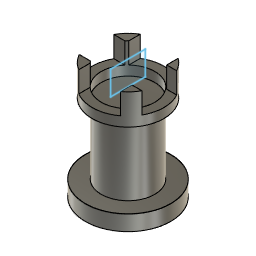
Rook v1 (Autodesk Fusion 360 design; units mm, degrees)
Autodesk Fusion 360 part; units mm, degrees
sketch "Sketch1" plane through (0, 0, 0) normal (0, 0, 1) x (1, 0, 0)
  circle A0 centre (0, 0) radius 27.94
  dimension "d1" = 55.88
  constraint coincident A0.centre origin
  measures "d1" diameter of A0
extrude "Extrude1" add sketch "Sketch1" along normal blind 10.16 makes body 1
sketch "Sketch2" plane through (0, 0, 0) normal (0, 0, 1) x (1, 0, 0)
  circle A0 centre (0, 0) radius 27.94
  dimension "d4" = 55.88
  constraint coincident A0.centre origin
  measures "d4" diameter of A0
extrude "Extrude2" add sketch "Sketch2" along normal blind 10 separate body makes body 2
sketch "Sketch3" plane through (0, 0, 10.16) normal (0, 0, 1) x (-1, 0, 0)
  circle A0 centre (0, 0) radius 27.94
  circle A1 centre (0, 0) radius 17.5
  dimension "d7" = 35
  constraint coincident A0.centre A1.centre
  measures "d7" diameter of A1
extrude "Extrude3" add sketch "Sketch3" along normal blind 46 contours A1 bodies 1
sketch "Sketch4" plane through (0, 0, 56.16) normal (0, 0, 1) x (-1, 0, 0)
  circle A0 centre (0, 0) radius 17.5
  circle A1 centre (0, 0) radius 23.5
  dimension "d10" = 47
  constraint coincident A0.centre A1.centre
  measures "d10" diameter of A1
extrude "Extrude4" add sketch "Sketch4" along normal blind 20 separate body makes body 3
sketch "Sketch5" plane through (0, 0, 0) normal (0, 1, 0) x (1, 0, 0)
  line L0 (-12.1078, -77.9552) -> (13.995, -77.9552)
  line L1 (13.995, -77.9552) -> (13.995, -62.4197)
  line L2 (13.995, -62.4197) -> (-12.1078, -62.4197)
  line L3 (-12.1078, -62.4197) -> (-12.1078, -77.9552)
  constraint horizontal L0
  constraint vertical L1
  constraint horizontal L2
  constraint vertical L3
extrude "Extrude5" cut sketch "Sketch5" against normal blind 80 bodies 3
extrude "Extrude6" cut sketch "Sketch5" along normal blind 45 bodies 3
sketch "Sketch6" plane through (0, 0, 0) normal (1, 0, 0) x (0, 1, 0)
  line L0 (-11.3774, 62.4072) -> (11.3148, 62.4072)
  line L1 (11.3148, 62.4072) -> (11.3148, 78.1358)
  line L2 (11.3148, 78.1358) -> (-11.3774, 78.1358)
  line L3 (-11.3774, 78.1358) -> (-11.3774, 62.4072)
  constraint horizontal L0
  constraint vertical L1
  constraint horizontal L2
  constraint vertical L3
extrude "Extrude7" cut sketch "Sketch6" against normal blind 32 bodies 3
extrude "Extrude8" cut sketch "Sketch6" along normal blind 33 bodies 3
